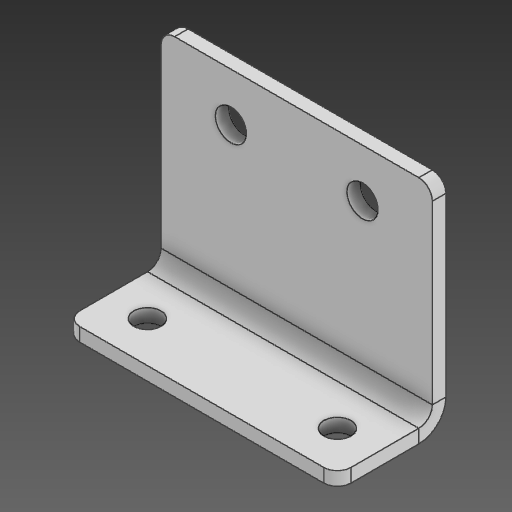
# Autodesk Inventor part: LimitSwitchMount
Saved by Autodesk Inventor 2025.2 (Build 292293000, 293)
## iProperties
Created: 2026-04-02
Part Number: LimitSwitchMount
Material: Generic
Document SubType Name: Sheet Metal
Designer: valer
Density: 1 g/cm^3
Sheet Metal Rule: Default_mm
Appearance: Default
Author: valer
Autodesk Inventor part; units mm, degrees
ref_plane "YZ Plane" through (0, 0, 0) normal (1, 0, 0) x (0, 1, 0)
ref_plane "XZ Plane" through (0, 0, 0) normal (0, 1, 0) x (-1, 0, 0)
ref_plane "XY Plane" through (0, 0, 0) normal (0, 0, 1) x (1, 0, 0)
sketch "Base" plane through (0, 0, 0) normal (0, 0, 1) x (1, 0, 0)
  line L0 (-10, -8) -> (10, -8)
  line L1 (10, -8) -> (10, 8)
  line L2 (10, 8) -> (-10, 8)
  line L3 (-10, 8) -> (-10, -8)
  line L4 (-10, -8) -> (10, 8) construction
  line L5 (10, -8) -> (-10, 8) construction
  point P0 (0, 0)
  dimension "d0" = 20
  dimension "d1" = 16
  measures "d0" distance of L1.end L2.end
  measures "d1" distance of L0.end L1.end
extrude "Plate1" add sketch "Base" along normal blind 1
sketch "Sketch2" plane through (10, -7, 0) normal (0, -1, 0) x (1, 0, 0)
  line L0 (-20, 0) -> (0, 0)
  line L1 (0, 0) -> (0, 8)
  line L2 (0, 8) -> (-20, 8)
  line L3 (-20, 8) -> (-20, 0)
  constraints: 6 end point, 1 horizontal, 1 perpendicular, 1 vertical
edge flange "MountFeature" height 8 angle 90 thickness 1 bend radius 1 thickness toward (0, -1, 0) relief tear relief width 1 relief depth 0.5 edges at (0, -8, 1) wall of the first edge with corners at (-10, -7, 0) (10, -7, 0) (10, -7, 8) (-10, -7, 8)
bend "Bend1"
corner "Corner1"
sketch "MountHoles" plane through (0, 0, 0) normal (0, 0, -1) x (-1, 0, 0)
  circle A0 centre (4.85, 4.448) radius 1.15 projected
  circle A1 centre (-4.85, 4.448) radius 1.15 projected
  point P0 (0, 0)
extrude "MountHolesFeature" cut sketch "MountHoles" against normal blind 1
fillet "EdgeFilletsFeature" radius 1 4 edges at (10, 8, 0.5) (-10, 8, 0.5) (-10, -7.5, 8) (10, -7.5, 8)
sketch "ArmMountHoles" plane through (-10, -8, 2) normal (0, -1, 0) x (1, 0, 0)
  line L0 (0, 3) -> (20, 3) construction
  line L1 (10, -3.8) -> (10, 8.8) construction
  circle A0 centre (3, 3) radius 1
  circle A1 centre (17, 3) radius 1
  line L2 (1, 6) -> (19, 6) projected
  line L3 (20, 0) -> (20, 5) projected
  line L4 (0, 0) -> (0, 5) projected
  point P0 (10, -2)
  dimension "d17" = 2
  dimension "d20" = 3
  constraints: 3 point on line, 2 centre point, 2 end point, 1 parallel, 1 symmetric about line, 1 other
  measures "d17" diameter of A0
  measures "d20" distance between parallel lines of L2 L0
extrude "ArmMountHolesFeature" cut sketch "ArmMountHoles" against normal blind 1
equation "\"d13\" = Thickness"
equation "\"d18\" = Thickness"
equation "\"d2\" = Thickness"
equation "\"d3\" = BendReliefWidth"
equation "\"d4\" = BendReliefDepth"
equation "\"d5\" = MinimumRemnant"
equation "\"d6\" = TransitionRadius"
equation "\"d9\" = BendRadius"
equation "\"d10\" = CornerReliefSize"
equation "\"d11\" = GapSize"
equation "\"d12\" = JacobiRadiusSize"
equation "\"BendRadius\" = Thickness"
equation "\"BendReliefWidth\" = Thickness"
equation "\"BendReliefDepth\" = 0.5 * Thickness"
equation "\"CornerReliefSize\" = 4 * Thickness"
equation "\"MinimumRemnant\" = 2 * Thickness"
equation "\"TransitionRadius\" = BendRadius"
equation "\"JacobiRadiusSize\" = BendRadius"
equation "\"GapSize\" = Thickness"
equation "\"Thickness\" = 1"
body "Solid1"
